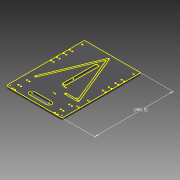
# Autodesk Inventor part: back board
Saved by Autodesk Inventor 2014 (Build 180170000, 170)
## iProperties
Created: 2013-07-23
Part Number: back board
Material: Generic
Document SubType Name: Modeling
Designer: employee
Density: 1 g/cm^3
Mass: 1788.17 g
Surface Area: 3314.84 cm^2
Volume: 1788.17 cm^3
Appearance: Gray
Author: employee
Autodesk Inventor part; units mm, degrees
ref_plane "YZ Plane" through (0, 0, 0) normal (1, 0, 0) x (0, 1, 0)
ref_plane "XZ Plane" through (0, 0, 0) normal (0, 1, 0) x (-1, 0, 0)
ref_plane "XY Plane" through (0, 0, 0) normal (0, 0, 1) x (1, 0, 0)
sketch "Sketch1" plane through (0, 0, 0) normal (0, 0, 1) x (1, 0, 0)
  line L0 (-165.5, 231.25) -> (165.5, 231.25)
  line L1 (165.5, 231.25) -> (165.5, -231.25)
  line L2 (165.5, -231.25) -> (-165.5, -231.25)
  line L3 (-165.5, -231.25) -> (-165.5, 231.25)
  point P0 (0, 0)
  point P1 (-165.5, 0)
  point P2 (0, 231.25)
  dimension "d0" = 331
  dimension "d2" = 462.5
  constraints: 8 end point, 2 midpoint, 2 parallel, 1 horizontal, 1 horizontal alignment, 1 perpendicular, 1 vertical alignment
  measures "d0" distance of L1.end L2.end
  measures "d2" distance of L0.end L1.end
extrude "Extrusion1" add sketch "Sketch1" along normal blind 12.5
fillet "Fillet1" radius 12.5 2 edges at (165.5, -231.25, 6.25) (-165.5, -231.25, 6.25)
sketch "Sketch6" plane through (0, 0, 12.5) normal (0, 0, 1) x (1, 0, 0)
  line L0 (165.5, 231.25) -> (-165.5, 231.25) projected
  line L1 (-10, 143.75) -> (10, 143.75)
  line L2 (10, 143.75) -> (10, -56.25)
  line L3 (10, -56.25) -> (-10, -56.25)
  line L4 (-10, -56.25) -> (-10, 143.75)
  point P0 (0, 0)
  point P1 (0, 143.75)
  dimension "d29" = 87.5
  dimension "d30" = 200
  dimension "d31" = 20
  dimension "d35" = 0
  constraints: 8 end point, 2 parallel, 1 horizontal, 1 midpoint, 1 perpendicular
  measures "d29" distance between parallel lines of L0 L1
  measures "d30" distance of L1.end L2.end
  measures "d31" distance of L1.start L1.end
  measures "d35" horizontal distance of point (0, 143.75) point (0, 0)
extrude "Extrusion6" cut sketch "Sketch6" against normal through all
fillet "Fillet2" radius 3 4 edges at (10, 143.75, 6.25) (-10, 143.75, 6.25) (-10, -56.25, 6.25) (10, -56.25, 6.25)
sketch "Sketch7" plane through (0, 0, 12.5) normal (0, 0, 1) x (1, 0, 0)
  line L0 (7, -56.25) -> (-7, -56.25) projected
  circle A0 centre (0, -61.25) radius 1.55
  point P0 (0, 0)
  point P1 (0, -56.25)
  dimension "d36" = 3.1
  dimension "d38" = 5
  constraints: 1 centre point, 1 midpoint, 1 vertical alignment
  measures "d36" diameter of A0
  measures "d38" distance of point (0, -56.25) A0.centre
extrude "Extrusion7" cut sketch "Sketch7" against normal through all
sketch "Sketch17" plane through (0, 0, 12.5) normal (0, 0, 1) x (1, 0, 0)
  line L0 (-141.9706, -92.134) -> (-108.0294, -92.134) projected
  line L1 (108.0294, -92.134) -> (141.9706, -92.134) projected
  circle A0 centre (125, -96.8965) radius 4.7625
  circle A1 centre (-125, -96.8965) radius 4.7625
  point P0 (0, 0)
  point P1 (125, -92.134)
  point P2 (-125, -92.134)
  dimension "d84" = 9.525
  constraints: 2 centre point, 2 midpoint, 2 tangent, 2 vertical alignment, 1 equal radius
  measures "d84" diameter of A1
extrude "Extrusion17" cut sketch "Sketch17" against normal through all
sketch "Sketch18" plane through (0, 0, 12.5) normal (0, 0, 1) x (1, 0, 0)
  circle A0 centre (125, -96.8965) radius 4.7625 projected
  circle A1 centre (-125, -96.8965) radius 4.7625 projected
  line L0 (-7, 143.75) -> (7, 143.75) projected
  line L1 (165.5, 231.25) -> (-165.5, 231.25) projected
  arc A2 (4.4029, 208.0655) -> (-4.4029, 208.0655) centre (0, 206.25) ccw
  line L2 (-4.4029, 208.0655) -> (-129.4029, -95.081)
  line L3 (-120.5971, -98.712) -> (0, 193.7568)
  line L4 (0, 193.7568) -> (120.5971, -98.712)
  line L5 (129.4029, -95.081) -> (4.4029, 208.0655)
  point P0 (0, 0)
  point P1 (0, 143.75)
  dimension "d88" = 25
  constraints: 8 end point, 7 point on circle, 6 tangent, 2 parallel, 1 centre point, 1 equal radius, 1 midpoint, 1 point on line, 1 vertical alignment
  measures "d88" distance from line of A2.centre L1
extrude "Extrusion18" cut sketch "Sketch18" against normal blind 6 contours A0 L4 L3 A1 L2 A2 L5
sketch "Sketch19" plane through (0, 0, 12.5) normal (0, 0, 1) x (1, 0, 0)
  arc A0 (120.5971, -98.712) -> (129.4029, -95.081) centre (125, -96.8965) ccw projected
  line L0 (120.5971, -98.712) -> (0, 193.7568) projected
  line L1 (51.616, -113.8671) -> (51.616, -79.9259) projected
  circle A1 centre (51.616, -96.8965) radius 4.7625
  line L2 (51.616, -101.659) -> (125, -101.659)
  line L3 (51.616, -92.134) -> (117.8847, -92.134)
  point P0 (0, 0)
  constraints: 4 end point, 3 point on circle, 3 point on line, 3 tangent, 1 centre point, 1 equal radius, 1 midpoint, 1 parallel
extrude "Extrusion19" cut sketch "Sketch19" against normal blind 4
fillet "Fillet14" radius 5 1 edges at (117.8847, -92.134, 10.5)
sketch "Sketch20" plane through (0, 0, 6.5) normal (0, 0, 1) x (1, 0, 0)
  arc A0 (4.4029, 208.0655) -> (-4.4029, 208.0655) centre (0, 206.25) ccw projected
  circle A1 centre (0, 206.25) radius 4.7625
  point P0 (0, 0)
  constraints: 1 centre point, 1 coincident, 1 concentric
extrude "Extrusion20" cut sketch "Sketch20" against normal through all
sketch "Sketch21" plane through (0, 0, 12.5) normal (0, 0, 1) x (1, 0, 0)
  arc A0 (145.5, 144.0161) -> (140.5, 139.0161) centre (145.5, 139.0161) ccw projected
  line L0 (140.5, 139.0161) -> (140.5, 29.0161) projected
  arc A1 (140.5, 29.0161) -> (145.5, 24.0161) centre (145.5, 29.0161) ccw projected
  line L1 (145.5, 24.0161) -> (160.5, 24.0161) projected
  arc A2 (160.5, 24.0161) -> (165.5, 29.0161) centre (160.5, 29.0161) ccw projected
  line L2 (165.5, 139.0161) -> (165.5, 29.0161) projected
  arc A3 (165.5, 139.0161) -> (160.5, 144.0161) centre (160.5, 139.0161) ccw projected
  line L3 (145.5, 144.0161) -> (160.5, 144.0161) projected
  circle A4 centre (160.5, 29.0161) radius 1.55 projected
  circle A5 centre (145.5, 64.0161) radius 1.55 projected
  circle A6 centre (160.5, 104.0161) radius 1.55 projected
  circle A7 centre (145.5, 139.0161) radius 1.55 projected
  circle A8 centre (160.5, 139.0161) radius 1.55 projected
  circle A9 centre (145.5, 104.0161) radius 1.55 projected
  circle A10 centre (160.5, 64.0161) radius 1.55 projected
  circle A11 centre (145.5, 29.0161) radius 1.55 projected
  arc A12 (-160.5, 144.0161) -> (-165.5, 139.0161) centre (-160.5, 139.0161) ccw projected
  line L4 (-165.5, 139.0161) -> (-165.5, 29.0161) projected
  arc A13 (-165.5, 29.0161) -> (-160.5, 24.0161) centre (-160.5, 29.0161) ccw projected
  line L5 (-160.5, 24.0161) -> (-145.5, 24.0161) projected
  arc A14 (-145.5, 24.0161) -> (-140.5, 29.0161) centre (-145.5, 29.0161) ccw projected
  line L6 (-140.5, 139.0161) -> (-140.5, 29.0161) projected
  arc A15 (-140.5, 139.0161) -> (-145.5, 144.0161) centre (-145.5, 139.0161) ccw projected
  line L7 (-160.5, 144.0161) -> (-145.5, 144.0161) projected
  circle A16 centre (-145.5, 29.0161) radius 1.55 projected
  circle A17 centre (-160.5, 64.0161) radius 1.55 projected
  circle A18 centre (-145.5, 104.0161) radius 1.55 projected
  circle A19 centre (-160.5, 139.0161) radius 1.55 projected
  circle A20 centre (-145.5, 139.0161) radius 1.55 projected
  circle A21 centre (-160.5, 104.0161) radius 1.55 projected
  circle A22 centre (-145.5, 64.0161) radius 1.55 projected
  circle A23 centre (-160.5, 29.0161) radius 1.55 projected
  arc A24 (-117.5, -231.25) -> (-112.5, -226.25) centre (-117.5, -226.25) ccw projected
  line L8 (-112.5, -136.25) -> (-112.5, -226.25) projected
  line L9 (-109, -136.25) -> (-112.5, -136.25) projected
  line L10 (-109, -131.25) -> (-109, -136.25) projected
  line L11 (-141, -131.25) -> (-109, -131.25) projected
  line L12 (-141, -136.25) -> (-141, -131.25) projected
  line L13 (-137.5, -136.25) -> (-141, -136.25) projected
  line L14 (-137.5, -136.25) -> (-137.5, -226.25) projected
  arc A25 (-137.5, -226.25) -> (-132.5, -231.25) centre (-132.5, -226.25) ccw projected
  line L15 (-117.5, -231.25) -> (-132.5, -231.25) projected
  circle A26 centre (-117.5, -141.25) radius 1.55 projected
  circle A27 centre (-132.5, -191.25) radius 1.55 projected
  circle A28 centre (-117.5, -226.25) radius 1.55 projected
  circle A29 centre (-132.5, -226.25) radius 1.55 projected
  circle A30 centre (-117.5, -191.25) radius 1.55 projected
  circle A31 centre (-132.5, -141.25) radius 1.55 projected
  arc A32 (132.5, -231.25) -> (137.5, -226.25) centre (132.5, -226.25) ccw projected
  line L16 (137.5, -136.25) -> (137.5, -226.25) projected
  line L17 (141, -136.25) -> (137.5, -136.25) projected
  line L18 (141, -131.25) -> (141, -136.25) projected
  line L19 (109, -131.25) -> (141, -131.25) projected
  line L20 (109, -136.25) -> (109, -131.25) projected
  line L21 (112.5, -136.25) -> (109, -136.25) projected
  line L22 (112.5, -136.25) -> (112.5, -226.25) projected
  arc A33 (112.5, -226.25) -> (117.5, -231.25) centre (117.5, -226.25) ccw projected
  line L23 (132.5, -231.25) -> (117.5, -231.25) projected
  circle A34 centre (132.5, -141.25) radius 1.55 projected
  circle A35 centre (117.5, -191.25) radius 1.55 projected
  circle A36 centre (132.5, -226.25) radius 1.55 projected
  circle A37 centre (117.5, -226.25) radius 1.55 projected
  circle A38 centre (132.5, -191.25) radius 1.55 projected
  circle A39 centre (117.5, -141.25) radius 1.55 projected
  arc A40 (22.5, -133.1465) -> (27.5, -128.1465) centre (22.5, -128.1465) ccw projected
  line L24 (12.5, -133.1465) -> (22.5, -133.1465) projected
  arc A41 (7.5, -128.1465) -> (12.5, -133.1465) centre (12.5, -128.1465) ccw projected
  line L25 (7.5, -128.1465) -> (7.5, -65.6465) projected
  arc A42 (12.5, -60.6465) -> (7.5, -65.6465) centre (12.5, -65.6465) ccw projected
  line L26 (22.5, -60.6465) -> (12.5, -60.6465) projected
  arc A43 (27.5, -65.6465) -> (22.5, -60.6465) centre (22.5, -65.6465) ccw projected
  line L27 (27.5, -65.6465) -> (27.5, -75.6465) projected
  line L28 (27.5, -75.6465) -> (12.5, -75.6465) projected
  line L29 (12.5, -75.6465) -> (12.5, -118.1465) projected
  line L30 (12.5, -118.1465) -> (27.5, -118.1465) projected
  line L31 (27.5, -118.1465) -> (27.5, -128.1465) projected
  circle A44 centre (22.5, -65.6465) radius 1.55 projected
  circle A45 centre (22.5, -128.1465) radius 1.55 projected
  circle A46 centre (12.5, -128.1465) radius 1.55 projected
  circle A47 centre (12.5, -65.6465) radius 1.55 projected
  arc A48 (160.5, -133.1465) -> (165.5, -128.1465) centre (160.5, -128.1465) ccw projected
  line L32 (150.5, -133.1465) -> (160.5, -133.1465) projected
  arc A49 (145.5, -128.1465) -> (150.5, -133.1465) centre (150.5, -128.1465) ccw projected
  line L33 (145.5, -105.1465) -> (145.5, -128.1465) projected
  line L34 (160.5, -105.1465) -> (145.5, -105.1465) projected
  line L35 (160.5, -75.6465) -> (160.5, -105.1465) projected
  line L36 (145.5, -75.6465) -> (160.5, -75.6465) projected
  line L37 (145.5, -75.6465) -> (145.5, -65.6465) projected
  arc A50 (150.5, -60.6465) -> (145.5, -65.6465) centre (150.5, -65.6465) ccw projected
  line L38 (160.5, -60.6465) -> (150.5, -60.6465) projected
  arc A51 (165.5, -65.6465) -> (160.5, -60.6465) centre (160.5, -65.6465) ccw projected
  line L39 (165.5, -65.6465) -> (165.5, -128.1465) projected
  circle A52 centre (160.5, -128.1465) radius 1.55 projected
  circle A53 centre (150.5, -65.6465) radius 1.55 projected
  circle A54 centre (160.5, -65.6465) radius 1.55 projected
  circle A55 centre (150.5, -128.1465) radius 1.55 projected
  circle A56 centre (-150.5, 203.75) radius 1.55 projected
  circle A57 centre (150.5, 203.75) radius 1.55 projected
  point P0 (0, 0)
extrude "Extrusion21" cut sketch "Sketch21" against normal through all contours A4 | A5 | A6 | A7 | A8 | A9 | A10 | A11 | A16 | A17 | A18 | A19 | A20 | A21 | A22 | A23 | A26 | A27 | A28 | A29 | A30 | A31 | A34 | A35 | A36 | A37 | A38 | A39 | A44 | A45 | A46 | A47 | A52 | A53 | A54 | A55 | A56 | A57
sketch "Sketch22" plane through (0, 0, 12.5) normal (0, 0, 1) x (1, 0, 0)
  circle A0 centre (-145.5, 64.0161) radius 1.55
  circle A1 centre (-145.5, 139.0161) radius 1.55
  circle A2 centre (-145.5, 104.0161) radius 1.55
  circle A3 centre (-145.5, 29.0161) radius 1.55
  circle A4 centre (160.5, 64.0161) radius 1.55
  circle A5 centre (160.5, 139.0161) radius 1.55
  circle A6 centre (160.5, 104.0161) radius 1.55
  circle A7 centre (160.5, 29.0161) radius 1.55
  circle A8 centre (132.5, -191.25) radius 1.55
  circle A9 centre (132.5, -226.25) radius 1.55
  circle A10 centre (132.5, -141.25) radius 1.55
  circle A11 centre (-117.5, -191.25) radius 1.55
  circle A12 centre (-117.5, -226.25) radius 1.55
  circle A13 centre (-117.5, -141.25) radius 1.55
  circle A14 centre (-132.5, -191.25) radius 1.55
  circle A15 centre (-132.5, -226.25) radius 1.55
  circle A16 centre (-132.5, -141.25) radius 1.55
  circle A17 centre (117.5, -191.25) radius 1.55
  circle A18 centre (117.5, -226.25) radius 1.55
  circle A19 centre (117.5, -141.25) radius 1.55
  circle A20 centre (145.5, 64.0161) radius 1.55
  circle A21 centre (145.5, 139.0161) radius 1.55
  circle A22 centre (145.5, 104.0161) radius 1.55
  circle A23 centre (145.5, 29.0161) radius 1.55
  circle A24 centre (-160.5, 64.0161) radius 1.55
  circle A25 centre (-160.5, 139.0161) radius 1.55
  circle A26 centre (-160.5, 104.0161) radius 1.55
  circle A27 centre (-160.5, 29.0161) radius 1.55
  circle A28 centre (-145.5, 64.0161) radius 1.55 projected
  circle A29 centre (-145.5, 139.0161) radius 1.55 projected
  circle A30 centre (-145.5, 104.0161) radius 1.55 projected
  circle A31 centre (-145.5, 29.0161) radius 1.55 projected
  circle A32 centre (160.5, 64.0161) radius 1.55 projected
  circle A33 centre (160.5, 139.0161) radius 1.55 projected
  circle A34 centre (160.5, 104.0161) radius 1.55 projected
  circle A35 centre (160.5, 29.0161) radius 1.55 projected
  circle A36 centre (132.5, -191.25) radius 1.55 projected
  circle A37 centre (132.5, -226.25) radius 1.55 projected
  circle A38 centre (132.5, -141.25) radius 1.55 projected
  circle A39 centre (-117.5, -191.25) radius 1.55 projected
  circle A40 centre (-117.5, -226.25) radius 1.55 projected
  circle A41 centre (-117.5, -141.25) radius 1.55 projected
  circle A42 centre (160.5, -65.6465) radius 1.55 projected
  circle A43 centre (160.5, -128.1465) radius 1.55 projected
  circle A44 centre (12.5, -128.1465) radius 1.55 projected
  circle A45 centre (22.5, -65.6465) radius 1.55 projected
  circle A46 centre (-150.5, 203.75) radius 1.55 projected
  circle A47 centre (150.5, 203.75) radius 1.55 projected
  circle A48 centre (22.5, -128.1465) radius 1.55 projected
  circle A49 centre (12.5, -65.6465) radius 1.55 projected
  circle A50 centre (150.5, -65.6465) radius 1.55 projected
  circle A51 centre (150.5, -128.1465) radius 1.55 projected
  circle A52 centre (-132.5, -191.25) radius 1.55 projected
  circle A53 centre (-132.5, -226.25) radius 1.55 projected
  circle A54 centre (-132.5, -141.25) radius 1.55 projected
  circle A55 centre (117.5, -191.25) radius 1.55 projected
  circle A56 centre (117.5, -226.25) radius 1.55 projected
  circle A57 centre (117.5, -141.25) radius 1.55 projected
  circle A58 centre (145.5, 64.0161) radius 1.55 projected
  circle A59 centre (145.5, 139.0161) radius 1.55 projected
  circle A60 centre (145.5, 104.0161) radius 1.55 projected
  circle A61 centre (145.5, 29.0161) radius 1.55 projected
  circle A62 centre (-160.5, 64.0161) radius 1.55 projected
  circle A63 centre (-160.5, 139.0161) radius 1.55 projected
  circle A64 centre (-160.5, 104.0161) radius 1.55 projected
  circle A65 centre (-160.5, 29.0161) radius 1.55 projected
  arc A66 (110.4146, -92.134) -> (115.0371, -85.228) centre (110.4146, -87.134) ccw projected
  line L0 (115.0371, -85.228) -> (0, 193.7568) projected
  line L1 (0, 193.7568) -> (-120.5971, -98.712) projected
  arc A67 (-129.4029, -95.081) -> (-120.5971, -98.712) centre (-125, -96.8965) ccw projected
  line L2 (-129.4029, -95.081) -> (-4.4029, 208.0655) projected
  arc A68 (4.4029, 208.0655) -> (-4.4029, 208.0655) centre (0, 206.25) ccw projected
  line L3 (4.4029, 208.0655) -> (129.4029, -95.081) projected
  arc A69 (125, -101.659) -> (129.4029, -95.081) centre (125, -96.8965) ccw projected
  line L4 (125, -101.659) -> (51.616, -101.659) projected
  arc A70 (51.616, -92.134) -> (51.616, -101.659) centre (51.616, -96.8965) ccw projected
  line L5 (51.616, -92.134) -> (110.4146, -92.134) projected
  circle A71 centre (0, -61.25) radius 1.55 projected
  line L6 (-10, -53.25) -> (-10, 140.75) projected
  arc A72 (-7, 143.75) -> (-10, 140.75) centre (-7, 140.75) ccw projected
  line L7 (-7, 143.75) -> (7, 143.75) projected
  arc A73 (10, 140.75) -> (7, 143.75) centre (7, 140.75) ccw projected
  line L8 (10, 140.75) -> (10, -53.25) projected
  arc A74 (7, -56.25) -> (10, -53.25) centre (7, -53.25) ccw projected
  line L9 (7, -56.25) -> (-7, -56.25) projected
  arc A75 (-10, -53.25) -> (-7, -56.25) centre (-7, -53.25) ccw projected
  arc A76 (-165.5, -218.75) -> (-153, -231.25) centre (-153, -218.75) ccw projected
  line L10 (-153, -231.25) -> (153, -231.25) projected
  arc A77 (153, -231.25) -> (165.5, -218.75) centre (153, -218.75) ccw projected
  line L11 (165.5, -218.75) -> (165.5, 231.25) projected
  line L12 (165.5, 231.25) -> (-165.5, 231.25) projected
  line L13 (-165.5, 231.25) -> (-165.5, -218.75) projected
  point P0 (0, 0)
  constraints: 28 centre point
hole "Hole1" at (145.5, 104.0161, 12.5) at (145.5, 139.0161, 12.5) at (160.5, 139.0161, 12.5) at (145.5, 29.0161, 12.5) at (160.5, 29.0161, 12.5) at (160.5, 64.0161, 12.5) at (145.5, 64.0161, 12.5) at (117.5, -141.25, 12.5) at (132.5, -141.25, 12.5) at (132.5, -191.25, 12.5) at (117.5, -191.25, 12.5) at (132.5, -226.25, 12.5) at (117.5, -226.25, 12.5) at (160.5, 104.0161, 12.5) at (-117.5, -141.25, 12.5) at (-117.5, -191.25, 12.5) at (-132.5, -141.25, 12.5) at (-132.5, -191.25, 12.5) at (-117.5, -226.25, 12.5) at (-132.5, -226.25, 12.5) at (-145.5, 29.0161, 12.5) at (-160.5, 139.0161, 12.5) at (-160.5, 64.0161, 12.5) at (-160.5, 29.0161, 12.5) at (-145.5, 64.0161, 12.5) at (-160.5, 104.0161, 12.5) at (-145.5, 104.0161, 12.5) at (-145.5, 139.0161, 12.5) at (-150.5, 203.75, 12.5) at (150.5, 203.75, 12.5) direction (0, 0, -1) diameter 3.4 end through all counterbore diameter 6.5 counterbore depth 3 clearance for "Socket Head Cap Screw" size "M3" standard "Ansi Metric M Profile"
sketch "Sketch23" plane through (0, 0, 0) normal (0, 0, -1) x (-1, 0, 0)
  line L0 (-153, -231.25) -> (153, -231.25) projected
  line L1 (62.5, -206.25) -> (-62.5, -206.25)
  line L2 (-62.5, -206.25) -> (-62.5, -181.25)
  line L3 (-62.5, -181.25) -> (62.5, -181.25)
  line L4 (62.5, -181.25) -> (62.5, -206.25)
  point P0 (0, 0)
  point P1 (0, -206.25)
  point P2 (0, -231.25)
  dimension "d106" = 25
  dimension "d107" = 125
  dimension "d108" = 25
  constraints: 8 end point, 2 midpoint, 2 parallel, 1 horizontal, 1 perpendicular, 1 vertical alignment
  measures "d106" distance between parallel lines of L0 L1
  measures "d107" distance of L1.start L1.end
  measures "d108" distance between parallel lines of L1 L3
extrude "Extrusion22" cut sketch "Sketch23" against normal through all
fillet "Fillet15" radius 12.5 4 edges at (-62.5, -181.25, 6.25) (62.5, -181.25, 6.25) (62.5, -206.25, 6.25) (-62.5, -206.25, 6.25)
fillet "Fillet17" radius 3 16 edges at (-58.8389, -184.9111, 0) (-58.8389, -202.5889, 0) (-62.5, -193.75, 0) (0, -206.25, 0) (62.5, -193.75, 0) (58.8389, -184.9111, 0) (58.8389, -202.5889, 0) (0, -181.25, 0) (62.5, -193.75, 12.5) (58.8389, -184.9111, 12.5) (58.8389, -202.5889, 12.5) (0, -206.25, 12.5) (-58.8389, -184.9111, 12.5) (-58.8389, -202.5889, 12.5) (-62.5, -193.75, 12.5) (0, -181.25, 12.5)
sketch "Sketch24" plane through (0, 0, 12.5) normal (0, 0, 1) x (1, 0, 0)
  arc A0 (-165.5, -218.75) -> (-153, -231.25) centre (-153, -218.75) ccw projected
  line L0 (-153, -231.25) -> (153, -231.25) projected
  arc A1 (153, -231.25) -> (165.5, -218.75) centre (153, -218.75) ccw projected
  line L1 (165.5, -218.75) -> (165.5, 231.25) projected
  line L2 (165.5, 231.25) -> (-165.5, 231.25) projected
  line L3 (-165.5, 231.25) -> (-165.5, -218.75) projected
  line L4 (-10, -53.25) -> (-10, 140.75) projected
  arc A2 (-7, 143.75) -> (-10, 140.75) centre (-7, 140.75) ccw projected
  line L5 (-7, 143.75) -> (7, 143.75) projected
  arc A3 (10, 140.75) -> (7, 143.75) centre (7, 140.75) ccw projected
  line L6 (10, 140.75) -> (10, -53.25) projected
  arc A4 (7, -56.25) -> (10, -53.25) centre (7, -53.25) ccw projected
  line L7 (7, -56.25) -> (-7, -56.25) projected
  arc A5 (-10, -53.25) -> (-7, -56.25) centre (-7, -53.25) ccw projected
  circle A6 centre (0, -61.25) radius 1.55 projected
  arc A7 (110.4146, -92.134) -> (115.0371, -85.228) centre (110.4146, -87.134) ccw projected
  line L8 (115.0371, -85.228) -> (0, 193.7568) projected
  line L9 (0, 193.7568) -> (-120.5971, -98.712) projected
  arc A8 (-129.4029, -95.081) -> (-120.5971, -98.712) centre (-125, -96.8965) ccw projected
  line L10 (-129.4029, -95.081) -> (-4.4029, 208.0655) projected
  arc A9 (4.4029, 208.0655) -> (-4.4029, 208.0655) centre (0, 206.25) ccw projected
  line L11 (4.4029, 208.0655) -> (129.4029, -95.081) projected
  arc A10 (125, -101.659) -> (129.4029, -95.081) centre (125, -96.8965) ccw projected
  line L12 (125, -101.659) -> (51.616, -101.659) projected
  arc A11 (51.616, -92.134) -> (51.616, -101.659) centre (51.616, -96.8965) ccw projected
  line L13 (51.616, -92.134) -> (110.4146, -92.134) projected
  circle A12 centre (150.5, -128.1465) radius 1.55 projected
  circle A13 centre (150.5, -65.6465) radius 1.55 projected
  circle A14 centre (12.5, -65.6465) radius 1.55 projected
  circle A15 centre (22.5, -128.1465) radius 1.55 projected
  circle A16 centre (22.5, -65.6465) radius 1.55 projected
  circle A17 centre (12.5, -128.1465) radius 1.55 projected
  circle A18 centre (160.5, -128.1465) radius 1.55 projected
  circle A19 centre (160.5, -65.6465) radius 1.55 projected
  circle A20 centre (150.5, 203.75) radius 3.25 projected
  circle A21 centre (-145.5, 139.0161) radius 3.25 projected
  circle A22 centre (-160.5, 104.0161) radius 3.25 projected
  circle A23 centre (-160.5, 29.0161) radius 3.25 projected
  circle A24 centre (-160.5, 139.0161) radius 3.25 projected
  circle A25 centre (-132.5, -226.25) radius 3.25 projected
  circle A26 centre (-132.5, -191.25) radius 3.25 projected
  circle A27 centre (-117.5, -191.25) radius 3.25 projected
  circle A28 centre (160.5, 104.0161) radius 3.25 projected
  circle A29 centre (132.5, -226.25) radius 3.25 projected
  circle A30 centre (132.5, -191.25) radius 3.25 projected
  circle A31 centre (117.5, -141.25) radius 3.25 projected
  circle A32 centre (160.5, 64.0161) radius 3.25 projected
  circle A33 centre (145.5, 29.0161) radius 3.25 projected
  circle A34 centre (145.5, 139.0161) radius 3.25 projected
  circle A35 centre (145.5, 104.0161) radius 3.25 projected
  circle A36 centre (160.5, 139.0161) radius 3.25 projected
  circle A37 centre (160.5, 29.0161) radius 3.25 projected
  circle A38 centre (145.5, 64.0161) radius 3.25 projected
  circle A39 centre (132.5, -141.25) radius 3.25 projected
  circle A40 centre (117.5, -191.25) radius 3.25 projected
  circle A41 centre (117.5, -226.25) radius 3.25 projected
  circle A42 centre (-117.5, -141.25) radius 3.25 projected
  circle A43 centre (-132.5, -141.25) radius 3.25 projected
  circle A44 centre (-117.5, -226.25) radius 3.25 projected
  circle A45 centre (-145.5, 29.0161) radius 3.25 projected
  circle A46 centre (-160.5, 64.0161) radius 3.25 projected
  circle A47 centre (-145.5, 64.0161) radius 3.25 projected
  circle A48 centre (-145.5, 104.0161) radius 3.25 projected
  circle A49 centre (-150.5, 203.75) radius 3.25 projected
  arc A50 (50, -209.25) -> (50, -178.25) centre (50, -193.75) ccw projected
  line L14 (-50, -209.25) -> (50, -209.25) projected
  arc A51 (-50, -178.25) -> (-50, -209.25) centre (-50, -193.75) ccw projected
  line L15 (50, -178.25) -> (-50, -178.25) projected
  point P0 (0, 0)
  dimension "d114" = 462.5
  measures "d114" distance between parallel lines of L0 L2
body "Solid1"
